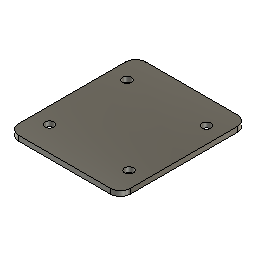
Mounting Plate v3 (Autodesk Fusion 360 design; units mm, degrees)
Autodesk Fusion 360 part; units mm, degrees
sketch "Sketch1" plane through (0, 0, 0) normal (0, 0, 1) x (1, 0, 0)
  line L0 (22, 25) -> (-22, 25)
  line L1 (-22, 25) -> (-22, -25)
  line L2 (-22, -25) -> (22, -25)
  line L3 (22, -25) -> (22, 25)
  line L4 (22, 25) -> (-22, -25) construction
  line L5 (-22, 25) -> (22, -25) construction
  line L6 (18.6, 18.6) -> (-18.6, 18.6)
  line L7 (-18.6, 18.6) -> (-18.6, -18.6)
  line L8 (-18.6, -18.6) -> (18.6, -18.6)
  line L9 (18.6, -18.6) -> (18.6, 18.6)
  line L10 (18.6, 18.6) -> (-18.6, -18.6) construction
  line L11 (-18.6, 18.6) -> (18.6, -18.6) construction
  line L12 (-18.6, 18.6) -> (-15.6272, 15.2218)
  circle A0 centre (-15.6272, 15.2218) radius 1.75
  line L13 (0, -25) -> (0, 25)
  line L14 (22, 0) -> (-22, 0)
  circle A1 centre (-15.6272, -15.2218) radius 1.75
  circle A2 centre (15.6272, -15.2218) radius 1.75
  circle A3 centre (15.6272, 15.2218) radius 1.75
  line L15 (-15.6272, 15.2218) -> (-18.6, 15.2218)
  line L16 (-18.6, 15.2218) -> (-22, 15.2218)
  line L17 (-18.8272, 15.2218) -> (-17.2272, 12.4505)
  line L18 (-17.2272, 12.4505) -> (-14.0272, 12.4505)
  line L19 (-14.0272, 12.4505) -> (-12.4272, 15.2218)
  line L20 (-12.4272, 15.2218) -> (-14.0272, 17.9931)
  line L21 (-14.0272, 17.9931) -> (-17.2272, 17.9931)
  line L22 (-17.2272, 17.9931) -> (-18.8272, 15.2218)
  line L23 (14.0272, 12.4505) -> (12.4272, 15.2218)
  line L24 (12.4272, 15.2218) -> (14.0272, 17.9931)
  line L25 (14.0272, 17.9931) -> (17.2272, 17.9931)
  line L26 (17.2272, 17.9931) -> (18.8272, 15.2218)
  line L27 (18.8272, 15.2218) -> (17.2272, 12.4505)
  line L28 (17.2272, 12.4505) -> (14.0272, 12.4505)
  line L29 (-14.0272, -17.9931) -> (-17.2272, -17.9931)
  line L30 (-17.2272, -17.9931) -> (-18.8272, -15.2218)
  line L31 (-12.4272, -15.2218) -> (-14.0272, -17.9931)
  line L32 (-14.0272, -12.4505) -> (-12.4272, -15.2218)
  line L33 (-17.2272, -12.4505) -> (-14.0272, -12.4505)
  line L34 (-18.8272, -15.2218) -> (-17.2272, -12.4505)
  line L35 (18.8272, -15.2218) -> (17.2272, -12.4505)
  line L36 (17.2272, -17.9931) -> (18.8272, -15.2218)
  line L37 (14.0272, -17.9931) -> (17.2272, -17.9931)
  line L38 (12.4272, -15.2218) -> (14.0272, -17.9931)
  line L39 (14.0272, -12.4505) -> (12.4272, -15.2218)
  line L40 (17.2272, -12.4505) -> (14.0272, -12.4505)
  point P0 (-15.6272, 15.2218)
  dimension "d1" = 44
  dimension "d2" = 50
  dimension "d3" = 37.2
  dimension "d4" = 37.2
  dimension "d5" = 4.5
  dimension "d6" = 3.5
  dimension "d11" = 3.2
  constraint horizontal L0
  constraint perpendicular L0 L1
  constraint parallel L0 L2
  constraint parallel L1 L3
  constraint coincident L4 origin
  constraint coincident L5 origin
  constraint horizontal L6
  constraint perpendicular L6 L7
  constraint parallel L6 L8
  constraint parallel L7 L9
  constraint coincident L10 origin
  constraint coincident L11 origin
  constraint parallel L5 L12
  constraint coincident P0 L12.end
  constraint midpoint L2 L13.start
  constraint midpoint L0 L13.end
  constraint midpoint L3 L14.start
  constraint midpoint L1 L14.end
  constraint symmetric A0 L14 A1
  constraint symmetric A0 L13 A3
  constraint symmetric L13 A1 A2
  constraint coincident L7 L15.end
  constraint perpendicular L7 L15
  constraint coincident L1 L16.end
  constraint perpendicular L1 L16
  constraint coincident L16 L17.start
  constraint symmetric L13 L17.start L26.end
  constraint symmetric L13 L17.end L27.end
  constraint symmetric L13 L18.end L23.start
  constraint symmetric L13 L19.end L23.end
  constraint symmetric L13 L20.end L24.end
  constraint symmetric L13 L21.end L25.end
  constraint symmetric L14 L17.start L30.end
  constraint symmetric L14 L17.end L33.start
  constraint symmetric L14 L18.end L32.start
  constraint symmetric L14 L19.end L31.start
  constraint symmetric L14 L20.end L29.start
  constraint symmetric L14 L21.end L29.end
  constraint symmetric L14 L23.start L39.start
  constraint symmetric L14 L23.end L38.start
  constraint symmetric L14 L24.end L37.start
  constraint symmetric L14 L25.end L36.start
  constraint symmetric L14 L26.end L35.start
  constraint symmetric L14 L27.end L35.end
  measures "d1" distance of L1.end L2.end
  measures "d2" distance of L0.end L1.end
  measures "d3" distance of L7.end L8.end
  measures "d4" distance of L6.end L7.end
  measures "d5" distance of L6.end P0
  measures "d6" diameter of A0
  measures "d11" distance of L17.start P0
extrude "Extrude1" add sketch "Sketch1" along normal blind 2 contours L0 L3 L6 L9 L13 L14 L26 L27 | L0 L1 L6 L7 L13 L16 L22 | L2 L3 L8 L9 L13 L14 L35 L36 | L6 L7 L12 L13 L14 L17 L18 L19 L20 L21 L22 | L6 L9 L13 L14 L23 L24 L25 L26 L27 L28 | L8 L9 L13 L14 L35 L36 L37 L38 L39 L40 | L1 L7 L14 L16 L17 | L7 L12 L22 | L7 L8 L13 L14 L29 L30 L31 L32 L33 L34 | L1 L2 L7 L8 L13 L14 L30 L34 | L9 L35 L36 | L9 L35 L36 L37 L38 L39 L40 | L9 L23 L24 L25 L26 L27 L28 | L9 L26 L27 | L7 L16 L22 | L7 L16 L17 | L7 L12 A0 L15 L22 | L7 L12 A0 L15 L17 L18 L19 L20 L21 L22 | L7 L29 L30 L31 L32 L33 L34 | L7 L30 L34
fillet "Fillet1" radius 4 4 edges at (22, -25, 1) (-22, -25, 1) (-22, 25, 1) (22, 25, 1)
